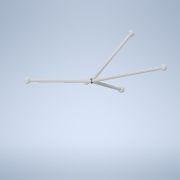
# Autodesk Inventor part: Coupler
Saved by Autodesk Inventor 2020.1 (Build 241239000, 239)
## iProperties
Created: 2019-10-25
Part Number: Coupler
Material: Generic
Document SubType Name: Modeling
Designer: sshel
Density: 1 g/cm^3
Appearance: Default
Mass: 190025 g
Surface Area: 74701 cm^2
Volume: 190025 cm^3
Author: sshel
Autodesk Inventor part; units mm, degrees
ref_plane "YZ Plane" through (0, 0, 0) normal (1, 0, 0) x (0, 1, 0)
ref_plane "XZ Plane" through (0, 0, 0) normal (0, 1, 0) x (-1, 0, 0)
ref_plane "XY Plane" through (0, 0, 0) normal (0, 0, 1) x (1, 0, 0)
ref_plane "Dyad1 plane" through (1360.64, 84.9394, -1028.14) normal (0.7968511, 0.0497443, -0.6021244) x (-0.0623048, 0.9980572, 0)
sketch "Sketch3" plane through (1360.64, 84.9394, -1028.14) normal (0.7968511, 0.0497443, -0.6021244) x (-0.0623048, 0.9980572, 0)
  circle A0 centre (0, 0) radius 50
  point P0 (0, 0)
  dimension "d16" = 50
  constraints: 1 centre point, 1 coincident
  measures "d16" radius of A0
sketch3d "import_point_3Dsketch"
  line L0 (1360.64, 84.9394, -1028.14) -> (0, 0, 0)
sweep "Dyad1 rod" add profiles "Sketch3" path "import_point_3Dsketch"
sketch "Sketch2" plane through (1360.64, 84.9394, -1028.14) normal (0.7968511, 0.0497443, -0.6021244) x (-0.0623048, 0.9980572, 0)
  circle A0 centre (0, 0) radius 100
  line L0 (100, 0) -> (-100, 0)
  point P0 (0, 0)
  dimension "d17" = 100
  constraints: 2 end point, 2 point on circle, 1 centre point, 1 coincident, 1 horizontal, 1 midpoint
  measures "d17" radius of A0
revolve "Dyad1 joint" add sketch "Sketch2" angle 360 about axis through (1354.4095, 184.7451, -1028.14) along (0.0623048, -0.9980572, 0) separate body picked at (-20.1483, -40.7644) contours A0 L0
ref_plane "Dyad2 plane" through (2143.42, -926.555, -102.536) normal (0.9170248, -0.3964104, -0.0438682) x (0.3967923, 0.9179084, 0)
sketch "Sketch4" plane through (2143.42, -926.555, -102.536) normal (0.9170248, -0.3964104, -0.0438682) x (0.3967923, 0.9179084, 0)
  circle A0 centre (0, 0) radius 50
  point P0 (0, 0)
  dimension "d14" = 50
  constraints: 1 centre point, 1 coincident
  measures "d14" radius of A0
sketch3d "import_point_3Dsketch for Dyad2 rod"
  line L0 (2143.42, -926.555, -102.536) -> (0, 0, 0)
sweep "Dyad2 rod" add profiles "Sketch4" path "import_point_3Dsketch for Dyad2 rod" separate body
sketch "Sketch5" plane through (2143.42, -926.555, -102.536) normal (0.9170248, -0.3964104, -0.0438682) x (0.3967923, 0.9179084, 0)
  circle A0 centre (0, 0) radius 100
  line L0 (100, 0) -> (-100, 0)
  point P0 (0, 0)
  dimension "d11" = 100
  constraints: 2 end point, 2 point on circle, 1 centre point, 1 coincident, 1 horizontal, 1 midpoint
  measures "d11" radius of A0
revolve "Dyad2 joint" add sketch "Sketch5" angle 360 about axis through (2183.0992, -834.7642, -102.536) along (-0.3967923, -0.9179084, 0) picked at (-20.1483, -40.7644) bodies 2 contours A0 L0
ref_plane "Dyad3 plane" through (1629.34, 1837.56, -1746.28) normal (0.5406896, 0.6097865, -0.5794956) x (-0.7482269, 0.6634429, 0)
sketch "Sketch6" plane through (1629.34, 1837.56, -1746.28) normal (0.5406896, 0.6097865, -0.5794956) x (-0.7482269, 0.6634429, 0)
  circle A0 centre (0, 0) radius 50
  point P0 (0, 0)
  dimension "d18" = 50
  constraints: 1 centre point, 1 coincident
  measures "d18" radius of A0
sketch3d "import_point_3Dsketch for Dyad3 rod"
  line L0 (1629.34, 1837.56, -1746.28) -> (0, 0, 0)
sweep "Dyad3 rod" add profiles "Sketch6" path "import_point_3Dsketch for Dyad3 rod" separate body
sketch "Sketch7" plane through (1629.34, 1837.56, -1746.28) normal (0.5406896, 0.6097865, -0.5794956) x (-0.7482269, 0.6634429, 0)
  circle A0 centre (0, 0) radius 100
  line L0 (100, 0) -> (-100, 0)
  point P0 (0, 0)
  dimension "d21" = 100
  constraints: 2 end point, 2 point on circle, 1 centre point, 1 coincident, 1 horizontal, 1 midpoint
  measures "d21" radius of A0
revolve "Dyad3 joint" add sketch "Sketch7" angle 360 about axis through (1554.5173, 1903.9043, -1746.28) along (0.7482269, -0.6634429, 0) picked at (-20.1483, -40.7644) bodies 2 contours A0 L0
ref_plane "Dyad4 plane" through (2357.47, 663.97, 245.527) normal (0.9577512, 0.269746, 0.0997484) x (-0.271098, 0.9625517, 0)
sketch "Sketch8" plane through (2357.47, 663.97, 245.527) normal (0.9577512, 0.269746, 0.0997484) x (-0.271098, 0.9625517, 0)
  circle A0 centre (0, 0) radius 50
  point P0 (0, 0)
  dimension "d23" = 50
  constraints: 1 centre point, 1 coincident
  measures "d23" radius of A0
sketch3d "import_point_3Dsketch for Dyad4 rod"
  line L0 (2357.47, 663.97, 245.527) -> (0, 0, 0)
sweep "Dyad4 rod" add profiles "Sketch8" path "import_point_3Dsketch for Dyad4 rod" separate body
sketch "Sketch9" plane through (2357.47, 663.97, 245.527) normal (0.9577512, 0.269746, 0.0997484) x (-0.271098, 0.9625517, 0)
  circle A0 centre (0, 0) radius 100
  line L0 (100, 0) -> (-100, 0)
  point P0 (0, 0)
  dimension "d26" = 100
  constraints: 2 end point, 2 point on circle, 1 centre point, 1 coincident, 1 horizontal, 1 midpoint
  measures "d26" radius of A0
revolve "Dyad4 joint" add sketch "Sketch9" angle 360 about axis through (2330.3602, 760.2252, 245.527) along (0.271098, -0.9625517, 0) picked at (-20.1483, -40.7644) bodies 2 contours A0 L0
ref_plane "Dyad5 plane" through (-1555.87, 1152.09, 232.757) normal (-0.7979116, 0.5908372, 0.119367) x (-0.595092, -0.8036576, 0)
sketch "Sketch10" plane through (-1555.87, 1152.09, 232.757) normal (-0.7979116, 0.5908372, 0.119367) x (-0.595092, -0.8036576, 0)
  circle A0 centre (0, 0) radius 50
  point P0 (0, 0)
  dimension "d28" = 50
  constraints: 1 centre point, 1 coincident
  measures "d28" radius of A0
sketch3d "import_point_3Dsketch for Dyad5 rod"
  line L0 (-1555.87, 1152.09, 232.757) -> (0, 0, 0)
sweep "Dyad5 rod" add profiles "Sketch10" path "import_point_3Dsketch for Dyad5 rod" separate body
sketch "Sketch11" plane through (-1555.87, 1152.09, 232.757) normal (-0.7979116, 0.5908372, 0.119367) x (-0.595092, -0.8036576, 0)
  circle A0 centre (0, 0) radius 100
  line L0 (100, 0) -> (-100, 0)
  point P0 (0, 0)
  dimension "d31" = 100
  constraints: 2 end point, 2 point on circle, 1 centre point, 1 coincident, 1 horizontal, 1 midpoint
  measures "d31" radius of A0
revolve "Dyad5 joint" add sketch "Sketch11" angle 360 about axis through (-1615.3792, 1071.7242, 232.757) along (0.595092, 0.8036576, 0) picked at (-20.1483, -40.7644) bodies 2 contours A0 L0
equation "\"d16\" = rod_radius"
equation "\"d17\" = S_radius"
equation "\"d14\" = rod_radius"
equation "\"d11\" = S_radius"
equation "\"d18\" = rod_radius"
equation "\"d21\" = S_radius"
equation "\"d23\" = rod_radius"
equation "\"d26\" = S_radius"
equation "\"d28\" = rod_radius"
equation "\"d31\" = S_radius"
equation "\"rod_radius\" = 50"
equation "\"S_radius\" = 2 * rod_radius"
body "Solid2"
body "Solid3"
body "Solid4"
body "Solid5"
body "Solid6"
body "Solid7"
